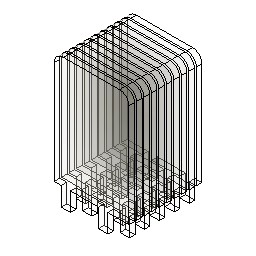
Digit (Autodesk Fusion 360 design; units mm, degrees)
Autodesk Fusion 360 part; units mm, degrees
sketch "Skizze1" plane through (0, 0, 0) normal (0, 0, 1) x (1, 0, 0) in component "Digit"
  line L0 (-15, 60) -> (15, 60)
  line L1 (20, 55) -> (20, 0)
  line L2 (-20, 55) -> (-20, 0)
  line L3 (-16.25, 0) -> (-16.25, -10)
  line L4 (-16.25, -10) -> (-11.25, -10)
  line L5 (-11.25, -10) -> (-11.25, 0)
  line L6 (3.75, 0) -> (3.75, -10)
  line L7 (3.75, -10) -> (8.75, -10)
  line L8 (8.75, -10) -> (8.75, 0)
  line L9 (-20, 0) -> (20, 0)
  arc A0 (-15, 60) -> (-20, 55) centre (-15, 55) ccw
  arc A1 (20, 55) -> (15, 60) centre (15, 55) ccw
  dimension "d5" = 5
  dimension "d6" = 5
  dimension "d8" = 10
  dimension "d9" = 5
  dimension "d10" = 5
  dimension "d11" = 60
  dimension "d12" = 40
  dimension "d16" = 3.75
  dimension "d18" = 15
  measures "d9" radius of A0
  measures "d10" radius of A1
  measures "d11" distance of L0 L9
  measures "d12" distance of L1 L2
  measures "d16" distance of L2 L3
  measures "d18" distance of L5 L6
extrude "Extrusion1" add sketch "Skizze1" along normal mid plane 3 in component "Digit"
pattern_linear "R-Anordnung1" [suppressed]
component "Digit" placed x (1, 0, 0) y (0, 0, 1) z (0, -1, 0) at (0, 0, 0)
component "Digit" placed x (-1, 0, 0) y (0, 0, 1) z (0, 1, 0) at (0, 4, 0)
component "Digit" placed x (1, 0, 0) y (0, 0, 1) z (0, -1, 0) at (0, 8, 0)
component "Digit" placed x (-1, 0, 0) y (0, 0, 1) z (0, 1, 0) at (0, 12, 0)
component "Digit" placed x (1, 0, 0) y (0, 0, 1) z (0, -1, 0) at (0, 16, 0)
component "Digit" placed x (-1, 0, 0) y (0, 0, 1) z (0, 1, 0) at (0, 20, 0)
component "Digit" placed x (1, 0, 0) y (0, 0, 1) z (0, -1, 0) at (0, 24, 0)
component "Digit" placed x (-1, 0, 0) y (0, 0, 1) z (0, 1, 0) at (0, 28, 0)
component "Digit" placed x (1, 0, 0) y (0, 0, 1) z (0, -1, 0) at (0, 32, 0)
component "Digit" placed x (-1, 0, 0) y (0, 0, 1) z (0, 1, 0) at (0, 36, 0)
equation "digit_width = 40 mm" comment "Width of acrylic digits"
equation "digit_height = 60 mm" comment "Height of acrylic digits"
equation "d5 = led_width"
equation "d6 = led_width"
equation "digit_thickness = 3 mm" comment "Thickness of acrylic digits"
equation "d9 = digit_roundness"
equation "d10 = digit_roundness"
equation "d11 = digit_height"
equation "d12 = digit_width"
equation "digit_roundness = 5 mm" comment "Roundness of acrylic digits (radius)"
equation "d14 = digit_thickness / 2"
equation "d16 = ( digit_width - 2 * led_width ) * 1 / 8"
equation "d18 = ( digit_width - 2 * led_width ) * 4 / 8"
equation "led_width = 5 mm" comment "Width and height of LEDs"
equation "d22 = digit_thickness + digit_spacing"
equation "digit_spacing = 1 mm" comment "Spacing of acrylic digits"
